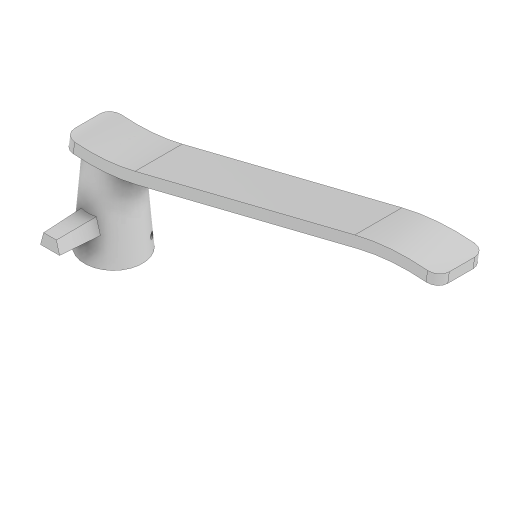
# Autodesk Inventor part: Part031.Window handle
Saved by Autodesk Inventor 2023.2 (Build 272271030, 271C)
## iProperties
Created: 2023-11-03
Part Number: Part031.Window handle
Material: Aluminum 6061-AHC
Document SubType Name: Modeling
Designer: User
Mass: 151.167 g
Surface Area: 208.117 cm^2
Volume: 55.9877 cm^3
Density: 2.7 g/cm^3
Appearance: Aluminum - Dark
Author: User
Autodesk Inventor part; units mm, degrees
ref_plane "YZ Plane" through (0, 0, 0) normal (1, 0, 0) x (0, 1, 0)
sketch "Sketch1" plane through (0, 0, 0) normal (0, 0, 1) x (1, 0, 0)
  arc A0 (-15.1699, 1.0608) -> (26.3695, 3.2378) centre (0, 109) ccw
  line L0 (26.3695, 3.2378) -> (147.6565, 33.478)
  arc A1 (191.4824, 35.7748) -> (147.6565, 33.478) centre (175.4775, -78.106) ccw
  arc A2 (192.3174, 41.7164) -> (146.2049, 39.2998) centre (175.4775, -78.106) ccw
  line L1 (146.2049, 39.2998) -> (24.918, 9.0595)
  arc A3 (-14.3348, 7.0024) -> (24.918, 9.0595) centre (0, 109) ccw
  line L2 (0, 109) -> (-15.1699, 1.0608) construction
  line L3 (0, 109) -> (26.3695, 3.2378) construction
  line L4 (0, 109) -> (0, 0) construction
  line L5 (175.4775, -78.106) -> (192.3174, 41.7164) construction
  line L6 (-14.3348, 7.0024) -> (-15.1699, 1.0608)
  line L7 (192.3174, 41.7164) -> (191.4824, 35.7748)
  line L8 (147.6565, 33.478) -> (175.4775, -78.106) construction
  point P0 (0, 0)
  dimension "d3" = 6
  dimension "d4" = 8
  dimension "d5" = 22
  dimension "d7" = 109
  dimension "d8" = 125
  dimension "d9" = 115
  dimension "d10" = 22
  dimension "d11" = 109
  constraints: 18 end point, 9 point on circle, 4 centre point, 4 tangent, 2 point on line, 1 collinear, 1 perpendicular, 1 vertical, 1 vertical alignment
  measures "d3" distance between parallel lines of L0 L1
  measures "d4" angle of L4 L2
  measures "d5" angle of L3 L2
  measures "d7" radius of A0
  measures "d8" distance of L0.start L0.end
  measures "d9" radius of A1
  measures "d10" angle of L8 L5
  measures "d11" distance of point (0, 0) L2.start
extrude "Extrusion1" add sketch "Sketch1" along normal mid plane 26
fillet "Fillet1" radius 6 4 edges at (-14.7523, 4.0316, 13) (-14.7523, 4.0316, -13) (191.8999, 38.7456, -13) (191.8999, 38.7456, 13)
ref_plane "Work Plane1" through (0, -46, 0) normal (0, 1, 0) x (-1, 0, 0)
sketch "Sketch2" plane through (0, -46, 0) normal (0, 1, 0) x (-1, 0, 0)
  circle A0 centre (0, 0) radius 16
  dimension "d16" = 32
  constraints: 1 centre point, 1 coincident
  measures "d16" diameter of A0
extrude "Extrusion2" add sketch "Sketch2" along normal up to next draft -4.5
ref_plane "Work Plane2" through (0, 0, 35) normal (0, 0, 1) x (1, 0, 0)
sketch "Sketch3" plane through (0, 0, 35) normal (0, 0, 1) x (1, 0, 0)
  line L0 (-5.25, -30) -> (-3.5083, -23.5)
  line L1 (-3.5083, -23.5) -> (3.5083, -23.5)
  line L2 (3.5083, -23.5) -> (5.25, -30)
  line L3 (5.25, -30) -> (-5.25, -30)
  line L4 (16, -46) -> (-16, -46) projected
  point P0 (0, 0)
  point P1 (0, -30)
  dimension "d20" = 10.5
  dimension "d21" = 30
  dimension "d22" = 16
  dimension "d23" = 6.5
  constraints: 8 end point, 1 equal length, 1 horizontal, 1 midpoint, 1 parallel, 1 vertical alignment
  measures "d20" distance of L2.end L0.start
  measures "d21" angle of L2 L0
  measures "d22" distance between parallel lines of L4 L3
  measures "d23" distance between parallel lines of L3 L1
extrude "Extrusion3" add sketch "Sketch3" against normal up to next draft 2
sketch "Sketch4" plane through (0, -46, 0) normal (0, -1, 0) x (1, 0, 0)
  circle A0 centre (0, 0) radius 16 projected
  constraints: 1 coincident
hole "Hole1" at (0, -46, 0) direction (0, 1, 0) diameter 16 depth 35 tip angle 118
sketch "Sketch5" plane through (0, 0, 0) normal (1, 0, 0) x (0, 1, 0)
  circle A0 centre (-38, -8) radius 1.5
  line L0 (-11, -8) -> (-46, -8) projected
  point P0 (0, 0)
  dimension "d33" = 3
  dimension "d34" = 8
  constraints: 1 centre point, 1 point on line
  measures "d33" diameter of A0
  measures "d34" distance of L0.end A0.centre
extrude "Extrusion4" cut sketch "Sketch5" along normal through all both and the other way through all
equation "\"d11\" = d7"
body "Solid1"
